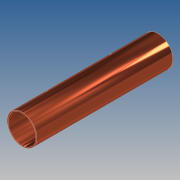
# Autodesk Inventor part: 2207_Cu Tube_V1
Saved by Autodesk Inventor 2020 (Build 240168000, 168)
## iProperties
Created: 2019-11-07
Part Number: 2207_Cu Tube_V1
Material: Generic
Document SubType Name: Modeling
Designer: RFLab
Density: 1 g/cm^3
Appearance: Default
Author: RFLab
Autodesk Inventor part; units mm, degrees
ref_plane "YZ Plane" through (0, 0, 0) normal (1, 0, 0) x (0, 1, 0)
ref_plane "XZ Plane" through (0, 0, 0) normal (0, 1, 0) x (-1, 0, 0)
ref_plane "XY Plane" through (0, 0, 0) normal (0, 0, 1) x (1, 0, 0)
sketch "Sketch1" plane through (0, 0, 0) normal (0, 0, 1) x (1, 0, 0)
  circle A0 centre (0, 0) radius 27
  dimension "d0" = 54
  constraints: 1 centre point, 1 coincident
  measures "d0" diameter of A0
extrude "Extrusion1" add sketch "Sketch1" along normal blind 246
sketch "Sketch2" plane through (0, 0, 246) normal (0, 0, 1) x (1, 0, 0)
  circle A0 centre (0, 0) radius 25.3
  dimension "d3" = 50.6
  constraints: 1 centre point, 1 coincident
  measures "d3" diameter of A0
extrude "Extrusion2" cut sketch "Sketch2" against normal through all
sketch "Sketch3" plane through (0, 0, 0) normal (0, 1, 0) x (-1, 0, 0)
  line L0 (0, 0) -> (0, 246)
  line L1 (0, 246) -> (0, 186)
  line L2 (0, 0) -> (0, 70)
  circle A0 centre (0, 186) radius 1.5
  circle A1 centre (0, 70) radius 1.5
  dimension "d6" = 60
  dimension "d7" = 246
  dimension "d8" = 70
  dimension "d9" = 3
  constraints: 6 end point, 2 centre point, 2 coincident, 2 point on line, 1 equal radius, 1 vertical
  measures "d6" distance of L1.end L0.end
  measures "d7" distance of L0.start L0.end
  measures "d8" distance of L2.end L0.start
  measures "d9" diameter of A1
extrude "Extrusion3" cut sketch "Sketch3" against normal through all
pattern_circular "Circular Pattern2" count 2 over 144 about axis through (0, 0, -10) along (0, 0, -1) of "Extrusion3"
body "Solid1"
